Autodesk Inventor part; units mm, degrees
(part 4 of 4)
  line L1499 (-9.3571, 29.0765) -> (-9.424, 29.0765) construction
  spline S459 degree 2 poles (-9.424, 29.0765) (-9.4797, 29.0765) (-9.5645, 29.1568) (-9.5645, 29.2103) knots 0 0 0 1 2 2 2
  line L1500 (-9.424, 29.0765) -> (-9.4797, 29.0765) construction
  line L1501 (-9.4797, 29.0765) -> (-9.5645, 29.1568) construction
  line L1502 (-9.5645, 29.1568) -> (-9.5645, 29.2103) construction
  spline S460 degree 2 poles (-9.5645, 29.2103) (-9.5645, 29.2505) (-9.54, 29.2862) knots 0 0 0 1 1 1
  line L1503 (-9.5645, 29.2103) -> (-9.5645, 29.2505) construction
  line L1504 (-9.5645, 29.2505) -> (-9.54, 29.2862) construction
  line L1505 (-9.54, 29.2862) -> (-9.1385, 29.8883)
  spline S461 degree 2 poles (-9.1385, 29.8883) (-9.3392, 29.9218) (-9.4574, 30.0801) knots 0 0 0 1 1 1
  line L1506 (-9.1385, 29.8883) -> (-9.3392, 29.9218) construction
  line L1507 (-9.3392, 29.9218) -> (-9.4574, 30.0801) construction
  spline S462 degree 2 poles (-9.4574, 30.0801) (-9.5623, 30.2229) (-9.5623, 30.4147) knots 0 0 0 1 1 1
  line L1508 (-9.4574, 30.0801) -> (-9.5623, 30.2229) construction
  line L1509 (-9.5623, 30.2229) -> (-9.5623, 30.4147) construction
  spline S463 degree 2 poles (-9.5623, 30.4147) (-9.5623, 30.631) (-9.4284, 30.7804) knots 0 0 0 1 1 1
  line L1510 (-9.5623, 30.4147) -> (-9.5623, 30.631) construction
  line L1511 (-9.5623, 30.631) -> (-9.4284, 30.7804) construction
  spline S464 degree 2 poles (-9.4284, 30.7804) (-9.2812, 30.9477) (-9.0292, 30.9477) knots 0 0 0 1 1 1
  line L1512 (-9.4284, 30.7804) -> (-9.2812, 30.9477) construction
  line L1513 (-9.2812, 30.9477) -> (-9.0292, 30.9477) construction
  line L1514 (-9.0292, 30.9477) -> (-8.3624, 30.9477)
  spline S465 degree 2 poles (-8.3624, 30.9477) (-8.2285, 30.9477) (-8.2285, 30.8139) knots 0 0 0 1 1 1
  line L1515 (-8.3624, 30.9477) -> (-8.2285, 30.9477) construction
  line L1516 (-8.2285, 30.9477) -> (-8.2285, 30.8139) construction
  line L1517 (-8.2285, 30.8139) -> (-8.2285, 29.2126)
  spline S466 degree 2 poles (-8.2285, 29.2126) (-8.2285, 29.0787) (-8.3624, 29.0787) knots 0 0 0 1 1 1
  line L1518 (-8.2285, 29.2126) -> (-8.2285, 29.0787) construction
  line L1519 (-8.2285, 29.0787) -> (-8.3624, 29.0787) construction
  spline S467 degree 2 poles (-8.3624, 29.0787) (-8.4962, 29.0787) (-8.4962, 29.2126) knots 0 0 0 1 1 1
  line L1520 (-8.3624, 29.0787) -> (-8.4962, 29.0787) construction
  line L1521 (-8.4962, 29.0787) -> (-8.4962, 29.2126) construction
  spline S468 degree 2 poles (-7.1602, 29.8794) (-7.2941, 29.8794) (-7.2941, 30.0132) knots 0 0 0 1 1 1
  line L1522 (-7.1602, 29.8794) -> (-7.2941, 29.8794) construction
  line L1523 (-7.2941, 29.8794) -> (-7.2941, 30.0132) construction
  spline S469 degree 2 poles (-7.2941, 30.0132) (-7.2941, 30.147) (-7.1602, 30.147) knots 0 0 0 1 1 1
  line L1524 (-7.2941, 30.0132) -> (-7.2941, 30.147) construction
  line L1525 (-7.2941, 30.147) -> (-7.1602, 30.147) construction
  line L1526 (-7.1602, 30.147) -> (-7.0264, 30.147)
  spline S470 degree 2 poles (-7.0264, 30.147) (-6.9015, 30.147) (-6.8279, 30.2296) knots 0 0 0 1 1 1
  line L1527 (-7.0264, 30.147) -> (-6.9015, 30.147) construction
  line L1528 (-6.9015, 30.147) -> (-6.8279, 30.2296) construction
  spline S471 degree 2 poles (-6.8279, 30.2296) (-6.761, 30.3054) (-6.761, 30.4147) knots 0 0 0 1 1 1
  line L1529 (-6.8279, 30.2296) -> (-6.761, 30.3054) construction
  line L1530 (-6.761, 30.3054) -> (-6.761, 30.4147) construction
  spline S472 degree 2 poles (-6.761, 30.4147) (-6.761, 30.524) (-6.8279, 30.5976) knots 0 0 0 1 1 1
  line L1531 (-6.761, 30.4147) -> (-6.761, 30.524) construction
  line L1532 (-6.761, 30.524) -> (-6.8279, 30.5976) construction
  spline S473 degree 2 poles (-6.8279, 30.5976) (-6.9015, 30.6801) (-7.0287, 30.6801) knots 0 0 0 1 1 1
  line L1533 (-6.8279, 30.5976) -> (-6.9015, 30.6801) construction
  line L1534 (-6.9015, 30.6801) -> (-7.0287, 30.6801) construction
  line L1535 (-7.0287, 30.6801) -> (-7.1625, 30.6801)
  spline S474 degree 2 poles (-7.1625, 30.6801) (-7.3431, 30.6801) (-7.4814, 30.573) knots 0 0 0 1 1 1
  line L1536 (-7.1625, 30.6801) -> (-7.3431, 30.6801) construction
  line L1537 (-7.3431, 30.6801) -> (-7.4814, 30.573) construction
  spline S475 degree 2 poles (-7.4814, 30.573) (-7.5215, 30.544) (-7.5639, 30.544) knots 0 0 0 1 1 1
  line L1538 (-7.4814, 30.573) -> (-7.5215, 30.544) construction
  line L1539 (-7.5215, 30.544) -> (-7.5639, 30.544) construction
  spline S476 degree 2 poles (-7.5639, 30.544) (-7.6175, 30.544) (-7.6977, 30.6266) (-7.6977, 30.6823) knots 0 0 0 1 2 2 2
  line L1540 (-7.5639, 30.544) -> (-7.6175, 30.544) construction
  line L1541 (-7.6175, 30.544) -> (-7.6977, 30.6266) construction
  line L1542 (-7.6977, 30.6266) -> (-7.6977, 30.6823) construction
  spline S477 degree 2 poles (-7.6977, 30.6823) (-7.6977, 30.7448) (-7.642, 30.7871) knots 0 0 0 1 1 1
  line L1543 (-7.6977, 30.6823) -> (-7.6977, 30.7448) construction
  line L1544 (-7.6977, 30.7448) -> (-7.642, 30.7871) construction
  spline S478 degree 2 poles (-7.642, 30.7871) (-7.4346, 30.9477) (-7.1625, 30.9477) knots 0 0 0 1 1 1
  line L1545 (-7.642, 30.7871) -> (-7.4346, 30.9477) construction
  line L1546 (-7.4346, 30.9477) -> (-7.1625, 30.9477) construction
  line L1547 (-7.1625, 30.9477) -> (-7.0287, 30.9477)
  spline S479 degree 2 poles (-7.0287, 30.9477) (-6.7766, 30.9477) (-6.6272, 30.7827) knots 0 0 0 1 1 1
  line L1548 (-7.0287, 30.9477) -> (-6.7766, 30.9477) construction
  line L1549 (-6.7766, 30.9477) -> (-6.6272, 30.7827) construction
  spline S480 degree 2 poles (-6.6272, 30.7827) (-6.4934, 30.631) (-6.4934, 30.4147) knots 0 0 0 1 1 1
  line L1550 (-6.6272, 30.7827) -> (-6.4934, 30.631) construction
  line L1551 (-6.4934, 30.631) -> (-6.4934, 30.4147) construction
  spline S481 degree 2 poles (-6.4934, 30.4147) (-6.4934, 30.1671) (-6.6607, 30.0132) knots 0 0 0 1 1 1
  line L1552 (-6.4934, 30.4147) -> (-6.4934, 30.1671) construction
  line L1553 (-6.4934, 30.1671) -> (-6.6607, 30.0132) construction
  spline S482 degree 2 poles (-6.6607, 30.0132) (-6.4934, 29.8593) (-6.4934, 29.6118) knots 0 0 0 1 1 1
  line L1554 (-6.6607, 30.0132) -> (-6.4934, 29.8593) construction
  line L1555 (-6.4934, 29.8593) -> (-6.4934, 29.6118) construction
  spline S483 degree 2 poles (-6.4934, 29.6118) (-6.4934, 29.3932) (-6.6272, 29.2438) knots 0 0 0 1 1 1
  line L1556 (-6.4934, 29.6118) -> (-6.4934, 29.3932) construction
  line L1557 (-6.4934, 29.3932) -> (-6.6272, 29.2438) construction
  spline S484 degree 2 poles (-6.6272, 29.2438) (-6.7766, 29.0787) (-7.0287, 29.0787) knots 0 0 0 1 1 1
  line L1558 (-6.6272, 29.2438) -> (-6.7766, 29.0787) construction
  line L1559 (-6.7766, 29.0787) -> (-7.0287, 29.0787) construction
  line L1560 (-7.0287, 29.0787) -> (-7.1625, 29.0787)
  spline S485 degree 2 poles (-7.1625, 29.0787) (-7.4346, 29.0787) (-7.642, 29.2393) knots 0 0 0 1 1 1
  line L1561 (-7.1625, 29.0787) -> (-7.4346, 29.0787) construction
  line L1562 (-7.4346, 29.0787) -> (-7.642, 29.2393) construction
  spline S486 degree 2 poles (-7.642, 29.2393) (-7.6977, 29.2817) (-7.6977, 29.3441) knots 0 0 0 1 1 1
  line L1563 (-7.642, 29.2393) -> (-7.6977, 29.2817) construction
  line L1564 (-7.6977, 29.2817) -> (-7.6977, 29.3441) construction
  spline S487 degree 2 poles (-7.6977, 29.3441) (-7.6977, 29.3999) (-7.6175, 29.4824) (-7.5639, 29.4824) knots 0 0 0 1 2 2 2
  line L1565 (-7.6977, 29.3441) -> (-7.6977, 29.3999) construction
  line L1566 (-7.6977, 29.3999) -> (-7.6175, 29.4824) construction
  line L1567 (-7.6175, 29.4824) -> (-7.5639, 29.4824) construction
  spline S488 degree 2 poles (-7.5639, 29.4824) (-7.5215, 29.4824) (-7.4814, 29.4534) knots 0 0 0 1 1 1
  line L1568 (-7.5639, 29.4824) -> (-7.5215, 29.4824) construction
  line L1569 (-7.5215, 29.4824) -> (-7.4814, 29.4534) construction
  spline S489 degree 2 poles (-7.4814, 29.4534) (-7.3431, 29.3464) (-7.1625, 29.3464) knots 0 0 0 1 1 1
  line L1570 (-7.4814, 29.4534) -> (-7.3431, 29.3464) construction
  line L1571 (-7.3431, 29.3464) -> (-7.1625, 29.3464) construction
  line L1572 (-7.1625, 29.3464) -> (-7.0287, 29.3464)
  spline S490 degree 2 poles (-7.0287, 29.3464) (-6.9015, 29.3464) (-6.8279, 29.4311) knots 0 0 0 1 1 1
  line L1573 (-7.0287, 29.3464) -> (-6.9015, 29.3464) construction
  line L1574 (-6.9015, 29.3464) -> (-6.8279, 29.4311) construction
  spline S491 degree 2 poles (-6.8279, 29.4311) (-6.761, 29.5069) (-6.761, 29.6162) knots 0 0 0 1 1 1
  line L1575 (-6.8279, 29.4311) -> (-6.761, 29.5069) construction
  line L1576 (-6.761, 29.5069) -> (-6.761, 29.6162) construction
  spline S492 degree 2 poles (-6.761, 29.6162) (-6.761, 29.8549) (-6.993, 29.8794) knots 0 0 0 1 1 1
  line L1577 (-6.761, 29.6162) -> (-6.761, 29.8549) construction
  line L1578 (-6.761, 29.8549) -> (-6.993, 29.8794) construction
  line L1579 (-6.993, 29.8794) -> (-7.1602, 29.8794)
  circle A34 centre (36.8398, 6.276) radius 1.5
  circle A35 centre (29.2433, 30.4282) radius 1.5
  circle A36 centre (-5.5726, 40.6117) radius 1.5
  circle A37 centre (5.1417, 40.6117) radius 1.5
  circle A38 centre (2.0046, 47.4047) radius 1.5
  circle A39 centre (-0.292, -33.0943) radius 1.5
  circle A40 centre (35.4878, -31.9185) radius 1.5
  circle A41 centre (0.0461, -47.8325) radius 0.9643
  circle A42 centre (3.801, -45.6645) radius 1.8
  circle A43 centre (-3.7089, -50.0004) radius 0.9643
  circle A44 centre (8.9424, -26.2127) radius 1.5
  circle A45 centre (7.523, 47.4047) radius 1.5
  circle A46 centre (5.1417, 36.8617) radius 1.5
  circle A47 centre (-5.5726, 36.8617) radius 1.5
  circle A48 centre (36.8398, -3.7237) radius 1.5
  circle A49 centre (9.8408, -3.7237) radius 1.5
  circle A50 centre (21.2935, 25.7008) radius 1.5
  circle A51 centre (-10.9297, 36.8617) radius 1.5
  circle A52 centre (-0.2154, 36.8617) radius 1.5
  circle A53 centre (11.5703, 36.8617) radius 1.5
  circle A54 centre (-0.292, -26.2127) radius 1.5
  circle A55 centre (35.4878, -24.2716) radius 1.5
  circle A56 centre (-3.7089, -45.6645) radius 0.9643
  circle A57 centre (3.801, -50.0004) radius 0.9643
  circle A58 centre (0.0461, -52.1683) radius 0.9643
  circle A59 centre (0.0461, -43.4966) radius 0.9643
  circle A60 centre (8.9424, -33.0943) radius 1.5
  circle A61 centre (12.6945, 47.4047) radius 1.5
  circle A62 centre (11.5703, 40.6117) radius 1.5
  circle A63 centre (-0.2154, 40.6117) radius 1.5
  circle A64 centre (-10.9297, 40.6117) radius 1.5
  circle A65 centre (14.7355, 30.4282) radius 1.5
  circle A66 centre (9.8408, 6.276) radius 1.5
  circle A67 centre (16.6071, -57.5893) radius 0.8036
  circle A68 centre (-16.6071, -57.5893) radius 0.8036
  circle A69 centre (16.6071, 57.5893) radius 0.8036
  circle A70 centre (-16.6071, 57.5893) radius 0.8036
  line L1580 (-16.6071, -7.9473) -> (-2.4622, -7.9473)
  line L1581 (-2.4622, -7.9473) -> (-2.4622, -20.8059)
  line L1582 (-2.4622, -20.8059) -> (-16.6071, -20.8059)
  line L1583 (-16.6071, -20.8059) -> (-16.6071, -7.9473)
  line L1584 (16.7895, -7.9473) -> (21.4868, -7.9473)
  line L1585 (21.4868, -7.9473) -> (21.4868, -20.8059)
  line L1586 (21.4868, -20.8059) -> (16.7895, -20.8059)
  line L1587 (16.7895, -20.8059) -> (16.7895, -7.9473)
  line L1588 (25.6343, 18.0091) -> (32.6879, 18.0091)
  line L1589 (32.6879, 18.0091) -> (32.6879, 9.0759)
  line L1590 (32.6879, 9.0759) -> (25.6343, 9.0759)
  line L1591 (25.6343, 9.0759) -> (25.6343, 18.0091)
  line L1592 (-2.4622, -7.9473) -> (5.6688, -7.9473)
  line L1593 (5.6688, -7.9473) -> (5.6688, 11.8984)
  line L1594 (5.6688, 11.8984) -> (9.8408, 11.8984)
  line L1595 (9.8408, 11.8984) -> (9.8408, 33.5781)
  line L1596 (9.8408, 33.5781) -> (9.8408, 36.2437)
  line L1597 (9.8408, 36.2437) -> (36.8398, 36.2437)
  line L1598 (36.8398, 36.2437) -> (36.8398, 11.7054)
  line L1599 (36.8398, 11.7054) -> (41.507, 11.7054)
  line L1600 (41.507, 11.7054) -> (41.507, -16.8274)
  line L1601 (41.507, -16.8274) -> (41.507, -36.9197)
  line L1602 (41.507, -36.9197) -> (-6.0097, -36.9197)
  line L1603 (-6.0097, -36.9197) -> (-6.0097, -20.8059)
  point P0 (0, 0)
  dimension "d0" = 3
  dimension "d1" = 3
  dimension "d2" = 3
  dimension "d11" = 3
  dimension "d12" = 3
  dimension "d13" = 3
  dimension "d14" = 3
  dimension "d15" = 3
  dimension "d16" = 3
  dimension "d17" = 3
  dimension "d19" = 3
  dimension "d20" = 3
  dimension "d21" = 3
  constraints: 892 end point, 71 centre point, 64 point on circle, 11 perpendicular, 6 parallel, 5 horizontal, 2 vertical, 1 point on line, 1479 other
  measures "d0" diameter of A65
  measures "d1" diameter of A50
  measures "d2" diameter of A35
  measures "d11" diameter of A66
  measures "d12" diameter of A34
  measures "d13" diameter of A48
  measures "d14" diameter of A49
  measures "d15" diameter of A44
  measures "d16" diameter of A54
  measures "d17" diameter of A39
  measures "d19" diameter of A60
  measures "d20" diameter of A55
  measures "d21" diameter of A40
extrude "Выдавливание1" add sketch "Эскиз1" along normal blind 2 contours A65 L2 L1595 L217 A26 L216 L1597 L236 L1584 L1587 L1586 L1602 L104 A17 L103 L102 L101 A16 L100 L227 L228 L225 A39 L427 S66 S65 L432 L1212 S349 S348 L1217 S351 S350 L1603 S272 L992 S271 L1582 L1581 L1592 L1593 L1594 L230 L231 L232 L0 | L0 L1595 L2 A65 | L232 L231 L230 L1595 | L1595 L211 S253 S252 A23 L212 L1597 L216 A26 L217 | L1595 L1596 L14 A11 L13 L1597 L212 A23 L211 | L211 S252 S253 | L1596 L1597 A53 L13 A11 L14 | L1581 L1582 L1583 L1580 | L1597 L1598 L1599 L1600 L1601 L1602 L236 L1586 L1585 L1584 | L1584 L1585 L1586 L236 | L236 L1586 L1587 L1584 | L1597 A53 | S271 L992 S272 L1603 | L1602 L100 A16 L101 L102 L103 A17 L104 | L225 A39 L228 L227 L1602 | S350 S351 L1217 S348 S349 L1212 A39 | A39 L432 S65 S66 L427 | L47 A44 L505 S100 S101 | S92 S93 A44 | S109 S110 S111 S112 S113 L521 S105 L525 S106 L529 A44 L51 S103 L516 S104 L520 S102 | S102 L520 S104 L516 S103 L51 A44 | A54 S120 S114 | L54 S115 S116 S117 L554 A54 | A54 L164 S307 S308 | L1107 S314 L1110 S315 S316 L162 L163 A54 L159 L160 L161 | L161 L160 L159 A54 | S273 L1006 S275 L1002 S274 L158 L157 | L165 L166 L167 S321 L1134 S322 L1138 S323 L1142 S324 L168 L169 L170 S325 S326 L1150 S327 S328 | L171 L172 L173 S329 S330 L174 L175 S331 L1161 S332 S333 L176 L177 S334 L1169 S335 S336 L1174 S337 L178 L179 S338 S339 | L1007 S276 L1011 S277 L1015 S278 L1018 S279 S280 S281 S282 S283 S284 | S290 S289 S288 S287 S286 S285 L1032 | L1060 S294 L1056 S293 L1052 S292 L1048 S291 | S295 L1063 S296 L1067 S297 L1071 S298 S299 S300 S301 S302 S303 | L1130 S320 L1126 S319 L1122 S318 L1118 S317 | L1588 L1589 L1590 L1591 picked at (11.4077, 35.9032)
extrude "Выдавливание2" add sketch "Эскиз1" against normal blind 8 contours L1581 L1582 L1583 L1580 | L1584 L1585 L1586 L236 | L236 L1586 L1587 L1584 | L1588 L1589 L1590 L1591
